Autodesk Fusion 360 part; units mm, degrees
(part 2 of 2)
extrude "Extrude1'''''''" add sketch "Sketch1 (6)" against normal blind 5 separate body contours A8 L8 A9 L9 A10 L10 A11 L11 makes body 21 in component "top"
sketch "Sketch2 (5)" plane through (0, 0, -6.0115) normal (0, 0, -1) x (1, 0, 0) in component "top"
  arc A0 (-26.2247, -104.2866) -> (-22.2247, -108.2866) centre (-22.2247, -104.2866) ccw
  line L0 (-22.2247, -108.2866) -> (39.3533, -108.2866)
  arc A1 (39.3533, -108.2866) -> (43.3533, -104.2866) centre (39.3533, -104.2866) ccw
  line L1 (43.3533, -104.2866) -> (43.3533, -22.5166)
  arc A2 (43.3533, -22.5166) -> (39.3533, -18.5166) centre (39.3533, -22.5166) ccw
  line L2 (39.3533, -18.5166) -> (-22.2247, -18.5166)
  arc A3 (-22.2247, -18.5166) -> (-26.2247, -22.5166) centre (-22.2247, -22.5166) ccw
  line L3 (-26.2247, -22.5166) -> (-26.2247, -104.2866)
  line L4 (39.3533, -25.5166) -> (39.3533, -101.2866)
  arc A4 (36.3533, -104.2866) -> (39.3533, -101.2866) centre (36.3533, -101.2866) ccw
  line L5 (36.3533, -104.2866) -> (-19.2247, -104.2866)
  arc A5 (-22.2247, -101.2866) -> (-19.2247, -104.2866) centre (-19.2247, -101.2866) ccw
  line L6 (-22.2247, -101.2866) -> (-22.2247, -25.5166)
  arc A6 (-19.2247, -22.5166) -> (-22.2247, -25.5166) centre (-19.2247, -25.5166) ccw
  line L7 (-19.2247, -22.5166) -> (36.3533, -22.5166)
  arc A7 (39.3533, -25.5166) -> (36.3533, -22.5166) centre (36.3533, -25.5166) ccw
sketch "Sketch3 (3)" plane through (0, 0, -6.0115) normal (0, 0, -1) x (1, 0, 0) in component "top"
extrude "Extrude2'''''''" add sketch "Sketch2 (5)" along normal blind 5 contours A0 L0 A1 L1 A2 L2 A3 L3 | L4 A4 L5 A5 L6 A6 L7 A7 bodies 21 in component "top"
sketch "Sketch4 (2)" plane through (43.3533, 0, 0) normal (1, 0, 0) x (0, 1, 0)
  arc A0 (63.4016, 9.9885) -> (67.4016, 9.9885) centre (65.4016, 9.9885) ccw
  line L0 (63.4016, 9.9885) -> (63.4016, 33.9885)
  arc A1 (67.4016, 33.9885) -> (63.4016, 33.9885) centre (65.4016, 33.9885) ccw
  line L1 (67.4016, 33.9885) -> (67.4016, 9.9885)
  line L2 (32.5166, 9.9885) -> (32.5166, 33.9885)
  arc A2 (36.5166, 33.9885) -> (32.5166, 33.9885) centre (34.5166, 33.9885) ccw
  line L3 (36.5166, 33.9885) -> (36.5166, 9.9885)
  arc A3 (32.5166, 9.9885) -> (36.5166, 9.9885) centre (34.5166, 9.9885) ccw
  arc A4 (78.8441, 9.9885) -> (82.8441, 9.9885) centre (80.8441, 9.9885) ccw
  line L4 (78.8441, 9.9885) -> (78.8441, 33.9885)
  arc A5 (82.8441, 33.9885) -> (78.8441, 33.9885) centre (80.8441, 33.9885) ccw
  line L5 (82.8441, 33.9885) -> (82.8441, 9.9885)
  arc A6 (47.9591, 9.9885) -> (51.9591, 9.9885) centre (49.9591, 9.9885) ccw
  line L6 (47.9591, 9.9885) -> (47.9591, 33.9885)
  arc A7 (51.9591, 33.9885) -> (47.9591, 33.9885) centre (49.9591, 33.9885) ccw
  line L7 (51.9591, 33.9885) -> (51.9591, 9.9885)
  arc A8 (94.2866, 9.9885) -> (98.2866, 9.9885) centre (96.2866, 9.9885) ccw
  line L8 (94.2866, 9.9885) -> (94.2866, 33.9885)
  arc A9 (98.2866, 33.9885) -> (94.2866, 33.9885) centre (96.2866, 33.9885) ccw
  line L9 (98.2866, 33.9885) -> (98.2866, 9.9885)
  line L10 (104.2866, -6.0115) -> (104.2866, 43.9885)
  line L11 (104.2866, 43.9885) -> (22.5166, 43.9885)
  line L12 (22.5166, 43.9885) -> (22.5166, -6.0115)
  line L13 (22.5166, -6.0115) -> (104.2866, -6.0115)
  circle A10 centre (29.0166, -3.5115) radius 1.5
  line L14 (23.0166, -6.0115) -> (23.0166, -1.0115)
  line L15 (25.5166, -1.0115) -> (101.2866, -1.0115)
  line L16 (63.4016, -6.0115) -> (63.4016, -1.0115) construction
  circle A11 centre (97.7866, -3.5115) radius 1.5
  dimension "d236" = 3
  dimension "d237" = 6
  dimension "d238" = 2.5
  constraint midpoint L13 L16.start
  constraint midpoint L15 L16.end
  constraint symmetric A10 L16 A11
  measures "d236" diameter of A10
  measures "d237" distance of A10.centre L14
  measures "d238" distance of A10.centre L15
extrude "Extrude9'" cut sketch "Sketch4 (2)" against normal blind 90 contours A10 | A11 bodies 20 in component "box"
extrude "Extrude3''''''" cut sketch "Sketch4 (2)" against normal blind 90 contours A10 | A11 bodies 21 in component "top"
component "Feather HUZZAH ESP8266 v1" placed x (1, 0, 0) y (0, -1, 0) z (0, 0, -1) at (-21.1467, 34.7166, 31.9885)
component "2.4\" TFT Feather Wing Copy v1" placed x (0, -1, 0) y (1, 0, 0) z (0, 0, 1) at (-21.2247, 95.2866, 38.3885)
component "sensors" placed x (1, 0, 0) y (0, 1, 0) z (0, 0, 1) at (0, 0, -11.26)
component "pms5003" placed x (1, 0, 0) y (0, 1, 0) z (0, 0, 1) at (-20.2157, 96.2866, 1.0885)
component "screen-pms5003-joint" placed x (1, 0, 0) y (0, 1, 0) z (0, 0, 1) at (0, 0, 0)
component "box" placed x (1, 0, 0) y (0, 1, 0) z (0, 0, 1) at (0, 0, 0)
component "top" placed x (1, 0, 0) y (0, 1, 0) z (0, 0, 1) at (0, 0, 0)
component "jlink" placed x (1, 0, 0) y (0, 1, 0) z (0, 0, 1) at (0.2, -21, 0) in component "pms5003"
equation "d118 = ( 5.15 / 2 ) * 1 mm"
equation "d210 = 81.77 mm - 20 mm"
equation "d220 = 61.57 mm - 20 mm"
named bodies: "pcb", "header medium", "header long", "pushbutton", "microSD", "switch", "display", "Huzzah PCB", "usb", "wifi pcb", "wifi mod", "JST", "header 12-pin", "header 16-pin"
